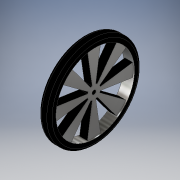
# Autodesk Inventor part: Wheel
Saved by Autodesk Inventor 2018 (Build 220112000, 112)
## iProperties
Created: 2018-02-19
Part Number: Wheel
Material: Generic
Document SubType Name: Modeling
Designer: Melda
Density: 1 g/cm^3
Appearance: Anodized - Black
Author: Melda
Autodesk Inventor part; units mm, degrees
ref_plane "YZ Plane" through (0, 0, 0) normal (1, 0, 0) x (0, 1, 0)
ref_plane "XZ Plane" through (0, 0, 0) normal (0, 1, 0) x (-1, 0, 0)
ref_plane "XY Plane" through (0, 0, 0) normal (0, 0, 1) x (1, 0, 0)
sketch "Sketch1" plane through (0, 0, 0) normal (1, 0, 0) x (0, 1, 0)
  circle A0 centre (0, 0) radius 35
  line L0 (29.5804, -5) -> (4.8166, -1.3417)
  line L1 (36.6755, 0) -> (35, 0)
  line L2 (29.5804, 5) -> (4.8166, 1.3417)
  line L3 (17.381, 24.452) -> (2.4572, 4.3546)
  line L4 (24.452, 17.381) -> (4.3546, 2.4572)
  line L5 (-5, 29.5804) -> (-1.3417, 4.8166)
  line L6 (5, 29.5804) -> (1.3417, 4.8166)
  line L7 (-24.452, 17.381) -> (-4.3546, 2.4572)
  line L8 (-17.381, 24.452) -> (-2.4572, 4.3546)
  line L9 (-29.5804, -5) -> (-4.8166, -1.3417)
  line L10 (-29.5804, 5) -> (-4.8166, 1.3417)
  line L11 (-17.381, -24.452) -> (-2.4572, -4.3546)
  line L12 (-24.452, -17.381) -> (-4.3546, -2.4572)
  line L13 (5, -29.5804) -> (1.3417, -4.8166)
  line L14 (-5, -29.5804) -> (-1.3417, -4.8166)
  line L15 (24.452, -17.381) -> (4.3546, -2.4572)
  line L16 (17.381, -24.452) -> (2.4572, -4.3546)
  arc A1 (4.8166, 1.3417) -> (4.3546, 2.4572) centre (0, 0) ccw
  arc A2 (2.4572, 4.3546) -> (1.3417, 4.8166) centre (0, 0) ccw
  arc A3 (-1.3417, 4.8166) -> (-2.4572, 4.3546) centre (0, 0) ccw
  arc A4 (-4.3546, 2.4572) -> (-4.8166, 1.3417) centre (0, 0) ccw
  arc A5 (-4.8166, -1.3417) -> (-4.3546, -2.4572) centre (0, 0) ccw
  arc A6 (-2.4572, -4.3546) -> (-1.3417, -4.8166) centre (0, 0) ccw
  arc A7 (1.3417, -4.8166) -> (2.4572, -4.3546) centre (0, 0) ccw
  arc A8 (4.3546, -2.4572) -> (4.8166, -1.3417) centre (0, 0) ccw
  arc A9 (29.5804, 5) -> (24.452, 17.381) centre (0, 0) ccw
  arc A10 (24.452, -17.381) -> (29.5804, -5) centre (0, 0) ccw
  arc A11 (5, -29.5804) -> (17.381, -24.452) centre (0, 0) ccw
  arc A12 (-17.381, -24.452) -> (-5, -29.5804) centre (0, 0) ccw
  arc A13 (-29.5804, -5) -> (-24.452, -17.381) centre (0, 0) ccw
  arc A14 (-24.452, 17.381) -> (-29.5804, 5) centre (0, 0) ccw
  arc A15 (17.381, 24.452) -> (5, 29.5804) centre (0, 0) ccw
  arc A16 (-5, 29.5804) -> (-17.381, 24.452) centre (0, 0) ccw
  dimension "d0" = 70
  constraints: 34 end point, 32 point on circle, 16 centre point, 3 coincident, 2 symmetric about line, 1 horizontal, 1 horizontal alignment, 51 other
extrude "Extrusion1" add sketch "Sketch1" along normal blind 8
sketch "Sketch2" plane through (8, 0, 0) normal (1, 0, 0) x (0, 0, -1)
  circle A0 centre (0, 0) radius 30
  dimension "d9" = 60
  constraints: 1 centre point, 1 coincident
  measures "d9" diameter of A0
extrude "Extrusion2" cut sketch "Sketch2" against normal blind 1
sketch "Sketch3" plane through (0, 0, 0) normal (-1, 0, 0) x (0, 0, 1)
  circle A0 centre (0, 0) radius 30
  constraints: 1 centre point, 1 coincident
extrude "Extrusion3" cut sketch "Sketch3" against normal blind 1
fillet "Fillet1" radius 2 2 edges at (0, -35, 0) (8, -35, 0)
sketch "Sketch4" plane through (1, 0, 0) normal (-1, 0, 0) x (0, 0, 1)
  circle A0 centre (0, 0) radius 1.5
  dimension "d15" = 3
  constraints: 1 centre point, 1 coincident
  measures "d15" diameter of A0
extrude "Extrusion4" cut sketch "Sketch4" against normal blind 10
body "Solid1"
